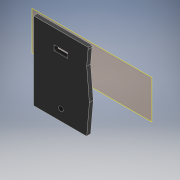
# Autodesk Inventor part: compnent box front L
Saved by Autodesk Inventor 2021 (Build 250183000, 183)
## iProperties
Created: 2023-01-12
Part Number: compnent box front L
Material: Generic
Document SubType Name: Modeling
Designer: boyle
Density: 1 g/cm^3
Appearance: Default
Author: boyle
Autodesk Inventor part; units mm, degrees
ref_plane "YZ Plane" through (0, 0, 0) normal (1, 0, 0) x (0, 1, 0)
ref_plane "XZ Plane" through (0, 0, 0) normal (0, 1, 0) x (-1, 0, 0)
ref_plane "XY Plane" through (0, 0, 0) normal (0, 0, 1) x (1, 0, 0)
ref_plane "Work Plane1" through (0, 0, 0) normal (0, 0, 1) x (1, 0, 0)
sketch "Sketch1" plane through (0, 0, 0) normal (0, 0, 1) x (1, 0, 0)
  line L0 (88.9, -98.425) -> (-88.9, -98.425)
  line L1 (-88.9, -98.425) -> (-88.9, -28.575)
  line L2 (-88.9, -28.575) -> (-88.9, 28.575)
  line L3 (-88.9, 28.575) -> (-85.09, 28.575)
  line L4 (88.9, 28.575) -> (88.9, -28.575)
  line L5 (85.09, 28.575) -> (88.9, 28.575)
  line L6 (88.9, -28.575) -> (88.9, -98.425)
  line L7 (-88.9, 28.575) -> (88.9, 28.575)
  line L8 (88.9, 28.575) -> (88.9, -98.425)
  line L9 (88.9, -98.425) -> (-88.9, -98.425)
  line L10 (-88.9, -98.425) -> (-88.9, 28.575)
  point P0 (0, 0)
extrude "Extrusion1" add sketch "Sketch1" along normal blind 6.35
sketch "Sketch2" plane through (0, 0, 6.35) normal (0, 0, 1) x (1, 0, 0)
  line L0 (-88.9, -98.425) -> (88.9, -98.425) projected
  line L1 (-88.9, -98.425) -> (-88.9, -28.575)
  line L2 (-88.9, 28.575) -> (-88.9, -98.425) projected
  line L3 (88.9, -98.425) -> (88.9, 28.575) projected
  circle A0 centre (-44.45, -80.9625) radius 3.8735
  line L4 (-88.9, 28.575) -> (88.9, 28.575)
  line L5 (88.9, 28.575) -> (88.9, -28.575)
  line L6 (88.9, -28.575) -> (-88.9, -28.575)
  line L7 (-88.9, -28.575) -> (-88.9, 28.575)
  line L8 (88.9, 28.575) -> (-88.9, 28.575) projected
  line L9 (0, 28.575) -> (0, -28.575)
  line L10 (-66.675, -80.9625) -> (-44.45, -80.9625)
  line L11 (-55.5874, 4.1336) -> (-33.3126, 4.1336)
  line L12 (-33.3126, 4.1336) -> (-33.3126, -4.1336)
  line L13 (-33.3126, -4.1336) -> (-55.5874, -4.1336)
  line L14 (-55.5874, -4.1336) -> (-55.5874, 4.1336)
  line L15 (-55.5874, 4.1336) -> (-33.3126, -4.1336) construction
  line L16 (-33.3126, 4.1336) -> (-55.5874, -4.1336) construction
  line L17 (34.3724, -7.1205) -> (54.0224, -7.1205)
  line L18 (54.0224, -7.1205) -> (54.0224, -24.6205)
  line L19 (54.0224, -24.6205) -> (34.3724, -24.6205)
  line L20 (34.3724, -24.6205) -> (34.3724, -7.1205)
  line L21 (34.3724, -7.1205) -> (54.0224, -24.6205) construction
  line L22 (54.0224, -7.1205) -> (34.3724, -24.6205) construction
  line L23 (39.4224, 16.9458) -> (54.0224, 16.9458)
  line L24 (54.0224, 16.9458) -> (54.0224, 0.5458)
  line L25 (54.0224, 0.5458) -> (39.4224, 0.5458)
  line L26 (39.4224, 0.5458) -> (39.4224, 16.9458)
  line L27 (39.4224, 16.9458) -> (54.0224, 0.5458) construction
  line L28 (54.0224, 16.9458) -> (39.4224, 0.5458) construction
  point P0 (0, 0)
  point P1 (44.1974, -15.8705)
  point P2 (46.7224, 8.7458)
  dimension "d2" = 69.85
  dimension "d5" = 7.747
  dimension "d8" = 22.2748
  dimension "d9" = 8.2672
  dimension "d10" = 16.4
  dimension "d11" = 14.6
  dimension "d12" = 19.65
  dimension "d13" = 17.5
  constraints: 50 end point, 8 parallel, 6 midpoint, 4 horizontal, 4 perpendicular, 2 point on line, 1 centre point
  measures "d2" distance of L0.start L1.end
  measures "d5" diameter of A0
  measures "d8" distance of L11.start L11.end
  measures "d9" distance of L11.end L12.end
  measures "d10" distance of L23.end L24.end
  measures "d11" distance of L23.start L23.end
  measures "d12" distance of L17.start L17.end
  measures "d13" distance of L17.end L18.end
extrude "Extrusion2" cut sketch "Sketch2" against normal through all contours A0 | L11 L12 L13 L14 | L17 L18 L19 L20 | L23 L24 L25 L26
sketch "Sketch3" plane through (0, 0, 6.35) normal (0, 0, 1) x (1, 0, 0)
  line L0 (54.0224, -7.1205) -> (54.0224, -24.6205) projected
  line L1 (54.0224, -24.6205) -> (34.3724, -24.6205) projected
  line L2 (34.3724, -24.6205) -> (34.3724, -7.1205) projected
  line L3 (34.3724, -7.1205) -> (54.0224, -7.1205) projected
  line L4 (39.4224, 0.5458) -> (39.4224, 16.9458) projected
  line L5 (39.4224, 16.9458) -> (54.0224, 16.9458) projected
  line L6 (54.0224, 16.9458) -> (54.0224, 0.5458) projected
  line L7 (54.0224, 0.5458) -> (39.4224, 0.5458) projected
  line L8 (88.9, 28.575) -> (-88.9, 28.575) projected
  line L9 (-88.9, -98.425) -> (88.9, -98.425) projected
  line L10 (88.9, -98.425) -> (88.9, 28.575) projected
  line L11 (-88.9, -98.425) -> (88.9, -98.425) projected
  line L12 (0, 25.29) -> (30.48, 25.29) construction
  line L13 (0, 25.29) -> (-2.1566, 0.6394)
  line L14 (0, 25.29) -> (24.7447, 25.29) construction
  line L15 (-2.1566, 0.6394) -> (0, -24.0111)
  line L16 (0, -24.0111) -> (2.1566, -48.6616)
  line L17 (2.1566, -48.6616) -> (0, -73.3121)
  line L18 (0, -73.3121) -> (-2.1566, -97.9626)
  line L19 (0, 25.29) -> (0, 28.575)
  line L20 (-2.1566, -97.9626) -> (-2.1566, -98.425)
  point P0 (0, 0)
  dimension "d21" = 24.7447
  dimension "d22" = 95
  dimension "d23" = 24.7447
  dimension "d24" = 24.7447
  dimension "d25" = 180
  dimension "d26" = 24.7447
  dimension "d27" = 24.7447
  constraints: 18 end point, 2 horizontal, 2 point on line, 1 collinear, 1 equal length, 1 midpoint, 1 perpendicular
  measures "d21" distance of L12.start L13.end
  measures "d22" angle of L13 L14
  measures "d23" distance of L13.end L15.end
  measures "d24" distance of L15.end L16.end
  measures "d25" angle of L16 L15
  measures "d26" distance of L16.end L17.end
  measures "d27" distance of L17.end L18.end
extrude "Extrusion3" cut sketch "Sketch3" against normal blind 25.4
body "Solid1"
